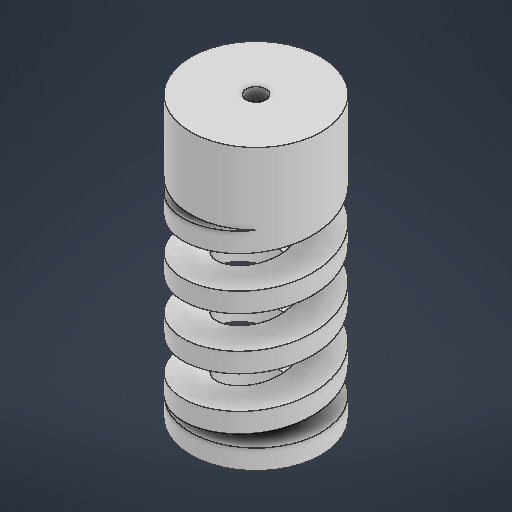
# Autodesk Inventor part: leg
Saved by Autodesk Inventor 2026.1 (Build 301233000, 233)
## iProperties
Created: 2026-05-24
Part Number: leg
Material: Generic
Document SubType Name: Modeling
Designer: emanuel
Density: 1 g/cm^3
Appearance: Default
Author: emanuel
Autodesk Inventor part; units mm, degrees
ref_plane "YZ Plane" through (0, 0, 0) normal (1, 0, 0) x (0, 1, 0)
ref_plane "XZ Plane" through (0, 0, 0) normal (0, 1, 0) x (-1, 0, 0)
ref_plane "XY Plane" through (0, 0, 0) normal (0, 0, 1) x (1, 0, 0)
sketch "Sketch1" plane through (0, 0, 0) normal (1, 0, 0) x (0, 1, 0)
  line L0 (0, 0) -> (0, -7.5)
  line L1 (-1.5, -5) -> (1.5, -5)
  line L2 (1.5, -5) -> (1.5, -10)
  line L3 (1.5, -10) -> (-1.5, -10)
  line L4 (-1.5, -10) -> (-1.5, -5)
  line L5 (-1.5, -5) -> (1.5, -10) construction
  line L6 (1.5, -5) -> (-1.5, -10) construction
  line L7 (0, 0) -> (4, 0)
  dimension "d0" = 7.5
  dimension "d1" = 3
  dimension "d2" = 5
  constraints: 16 end point, 2 horizontal, 2 midpoint, 2 parallel, 1 perpendicular, 1 vertical
  measures "d0" distance of L0.start L0.end
  measures "d1" distance of L2.end L3.end
  measures "d2" distance of L1.end L2.end
coil "Coil1" sketch "Sketch1" operation add axis through (0, 0, 0) along (0, 1, 0) pitch 8 turns 4 hand right
sketch "Sketch2" plane through (0, -1.5, -5) normal (1, 0, 0) x (0, 0, -1)
  line L0 (0, 3) -> (5, 3) projected
  line L1 (0, 0) -> (5, 0)
  line L2 (5, 0) -> (5, 3)
  line L3 (5, 3) -> (0, 3)
  line L4 (0, 3) -> (0, 0)
  line L5 (0, 0) -> (5, 3) construction
  line L6 (5, 0) -> (0, 3) construction
  line L7 (-5, 1.5) -> (-5, 3.786)
  point P0 (2.5, 1.5)
  dimension "d19" = 5
  constraints: 14 end point, 2 midpoint, 2 parallel, 1 horizontal, 1 perpendicular, 1 vertical
  measures "d19" distance of L1.start L1.end
revolve "Revolution1" add sketch "Sketch2" angle 360 about axis through (0, 0, 0) along (0, 1, 0)
sketch "Sketch3" plane through (0, 30.5, -5) normal (-1, 0, 0) x (0, 0, 1)
  line L0 (0, 3) -> (-5, 3) projected
  line L1 (-5, 3) -> (-2.5, 3)
  line L2 (-2.5, 3) -> (-2.5, 1.5)
  line L3 (-2.5, 1.5) -> (-5, 1.5)
  line L4 (-5, 1.5) -> (-5, 3)
  line L5 (0, 0) -> (-5, 0)
  line L6 (-5, 0) -> (-5, 3)
  line L7 (-5, 3) -> (0, 3)
  line L8 (0, 3) -> (0, 0)
  line L9 (0, 0) -> (-5, 3) construction
  line L10 (-5, 0) -> (0, 3) construction
  line L11 (-2.5, 1.5) -> (5, 1.5)
  line L12 (5, 1.5) -> (5, 8.6218)
  point P0 (5, -30.5)
  dimension "d12" = 2.5
  dimension "d13" = 1.5
  dimension "d14" = 7.5
  constraints: 24 end point, 4 parallel, 3 perpendicular, 2 horizontal, 2 midpoint, 1 point on line
  measures "d12" distance of L2.end L3.end
  measures "d13" distance of L1.end L2.end
  measures "d14" distance of L2.end L11.end
revolve "Revolution2" add sketch "Sketch3" angle 360 about axis through (0, 32, 0) along (0, 1, 0)
sketch "Sketch4" plane through (0, 33.5, 0) normal (0, 1, 0) x (1, 0, 0)
  circle A0 centre (0, 0) radius 1.5
  line L0 (0, 5) -> (0, 10) projected
  circle A1 centre (0, 0) radius 5
  point P0 (0, 0)
  dimension "d16" = 3
  constraints: 2 coincident, 1 centre point, 1 vertical alignment, 2 other
  measures "d16" diameter of A0
extrude "Extrusion1" add sketch "Sketch4" against normal blind 3
sketch "Sketch5" plane through (0, 33.5, 0) normal (0, 1, 0) x (1, 0, 0)
  circle A0 centre (0, 0) radius 1.5 projected
  circle A1 centre (0, 0) radius 1.5
  line L0 (0, 5) -> (0, 10) projected
  circle A2 centre (0, 0) radius 10
  point P0 (0, 0)
  constraints: 2 coincident, 1 centre point, 1 vertical alignment, 2 other
extrude "Extrusion2" add sketch "Sketch5" along normal blind 8
body "Solid1"
